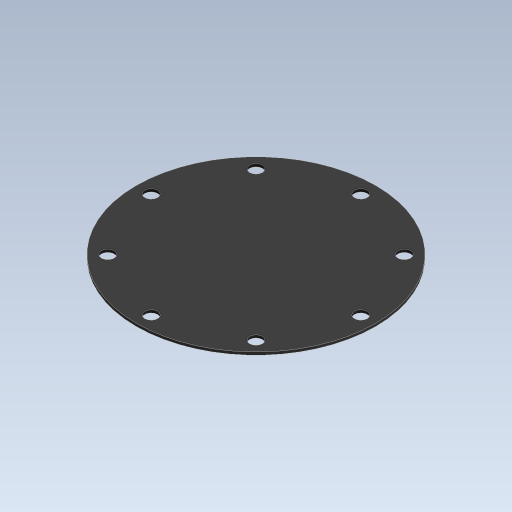
# Autodesk Inventor part: Pump-Motor-CW-Rotation:Diaphragm
Saved by Autodesk Inventor 2024.2 (Build 282272000, 272)
## iProperties
Created: 2025-06-16
Material: Rubber
Document SubType Name: Modeling
Designer: cw
Density: 0.93 g/cm^3
Appearance: Rubber - Black
Author: cw
Autodesk Inventor part; units mm, degrees
ref_plane "YZ Plane" through (0, 0, 0) normal (1, 0, 0) x (0, 1, 0)
ref_plane "XZ Plane" through (0, 0, 0) normal (0, 1, 0) x (-1, 0, 0)
ref_plane "XY Plane" through (0, 0, 0) normal (0, 0, 1) x (1, 0, 0)
sketch "Sketch1" plane through (0, 0, 0) normal (0, 0, 1) x (1, 0, 0)
  circle A0 centre (0, 0) radius 65
  dimension "d0" = 130
  constraints: 1 centre point, 1 coincident
  measures "d0" diameter of A0
extrude "Extrusion1" add sketch "Sketch1" along normal blind 1.5
sketch "Sketch2" plane through (0, 0, 1.5) normal (0, 0, 1) x (1, 0, 0)
  circle A0 centre (0, 0) radius 57 construction
  point P0 (-57, 0)
  dimension "d3" = 114
  constraints: 2 horizontal alignment, 1 coincident, 2 other
hole "Hole1" at (-57, 0, 1.5) direction (0, 0, -1) diameter 7 end through all
pattern_circular "Circular Pattern1" count 8 over 360 about axis through (0, 0, -10) along (0, 0, 1) of "Hole1"
body "Solid1"
